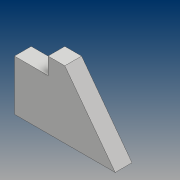
# Autodesk Inventor part: 43 (22000.000 mm^3)
Saved by Autodesk Inventor 2018 (Build 220112000, 112)
## iProperties
Created: 2020-09-18
Part Number: 43 (22000.000 mm^3)
Material: 一般
Document SubType Name: Modeling
Designer: 88697
Density: 1 g/cm^3
Appearance: 預設
Author: 88697
Autodesk Inventor part; units mm, degrees
ref_plane "YZ Plane" through (0, 0, 0) normal (1, 0, 0) x (0, 1, 0)
ref_plane "XZ Plane" through (0, 0, 0) normal (0, 1, 0) x (-1, 0, 0)
ref_plane "XY Plane" through (0, 0, 0) normal (0, 0, 1) x (1, 0, 0)
sketch "草圖1" plane through (0, 0, 0) normal (0, 1, 0) x (-1, 0, 0)
  line L0 (0, -10) -> (-20, -10)
  line L1 (-20, -10) -> (-20, 0)
  line L2 (-20, 0) -> (-30, 0)
  line L3 (-30, 0) -> (-60, -40)
  line L4 (-60, -40) -> (0, -40)
  line L5 (0, -40) -> (0, -10)
  point P0 (0, 0)
  dimension "d0" = 10
  dimension "d1" = 20
  dimension "d2" = 10
  dimension "d3" = 0
  dimension "d4" = 10
  dimension "d5" = 30
  dimension "d6" = 60
  constraints: 12 end point, 3 perpendicular, 1 horizontal, 1 parallel
  measures "d0" distance from line of L0 point (0, 0)
  measures "d1" distance from line of point (0, 0) L1
  measures "d2" distance of L1.end L2.end
  measures "d3" distance from line of L5 point (0, 0)
  measures "d4" distance between parallel lines of L2 L0
  measures "d5" distance of L4.end L0.start
  measures "d6" distance of L3.end L4.end
extrude "擠出1" add sketch "草圖1" along normal blind 10
sketch "草圖2" plane through (0, 0, -40) normal (-1, 0, 0) x (0, 0, 1)
  line L0 (40, 10) -> (0, 10) projected
  line L1 (0, 10) -> (0, 30)
  line L2 (0, 30) -> (20, 20)
  line L3 (20, 20) -> (20, 10)
  line L4 (20, 10) -> (0, 10)
  point P0 (40, 0)
  dimension "d9" = 20
  dimension "d10" = 20
  dimension "d11" = 10
  constraints: 8 end point, 1 collinear, 1 midpoint, 1 parallel, 1 vertical
  measures "d9" distance of L0.end L1.end
  measures "d10" distance between parallel lines of L1 L3
  measures "d11" distance of L2.end L3.end
extrude "擠出2" add sketch "草圖2" against normal blind 20
